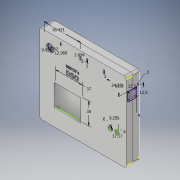
# Autodesk Inventor part: case
Saved by Autodesk Inventor 2019 (Build 230136000, 136)
## iProperties
Created: 2019-10-15
Part Number: case
Material: Generic
Document SubType Name: Modeling
Designer: Bill
Density: 1 g/cm^3
Appearance: Default
Author: Bill
Autodesk Inventor part; units mm, degrees
ref_plane "YZ Plane" through (0, 0, 0) normal (1, 0, 0) x (0, 1, 0)
ref_plane "XZ Plane" through (0, 0, 0) normal (0, 1, 0) x (-1, 0, 0)
ref_plane "XY Plane" through (0, 0, 0) normal (0, 0, 1) x (1, 0, 0)
sketch "Sketch1" plane through (0, 0, 0) normal (0, 0, 1) x (1, 0, 0)
  line L0 (0, 0) -> (110, 0) construction
  line L1 (110, 0) -> (110, 100) construction
  line L2 (110, 100) -> (0, 100) construction
  line L3 (0, 100) -> (0, 0) construction
  circle A0 centre (4, 96) radius 1.4
  circle A1 centre (106, 96) radius 1.4
  circle A2 centre (4, 4) radius 1.4
  circle A3 centre (106, 4) radius 1.4
  line L4 (-3, -3) -> (113, -3)
  line L5 (113, -3) -> (113, 103)
  line L6 (113, 103) -> (-3, 103)
  line L7 (-3, 103) -> (-3, -3)
  circle A4 centre (4, 96) radius 2
  circle A5 centre (106, 96) radius 2
  circle A6 centre (106, 4) radius 2
  circle A7 centre (4, 4) radius 2
  dimension "d0" = 100
  dimension "d1" = 110
  dimension "d2" = 2.8
  dimension "d3" = 2.8
  dimension "d4" = 2.8
  dimension "d5" = 2.8
  dimension "d6" = 4
  dimension "d7" = 4
  dimension "d8" = 4
  dimension "d9" = 4
  dimension "d10" = 4
  dimension "d11" = 4
  dimension "d12" = 4
  dimension "d13" = 4
  dimension "d14" = 3
  dimension "d27" = 4
  dimension "d28" = 4
  constraints: 16 end point, 8 centre point, 4 coincident, 4 parallel, 2 perpendicular, 1 horizontal, 3 other
  measures "d0" distance between parallel lines of L0 L2
  measures "d1" distance between parallel lines of L1 L3
  measures "d2" diameter of A0
  measures "d3" diameter of A1
  measures "d4" diameter of A2
  measures "d5" diameter of A3
  measures "d6" distance from line of L3 A0.centre
  measures "d7" distance from line of L2 A0.centre
  measures "d8" distance from line of A1.centre L2
  measures "d9" distance from line of L1 A1.centre
  measures "d10" distance from line of L3 A2.centre
  measures "d11" distance from line of L0 A2.centre
  measures "d12" distance from line of L1 A3.centre
  measures "d13" distance from line of L0 A3.centre
  measures "d14" distance between parallel lines of L3 L7
  measures "d27" diameter of A4
  measures "d28" diameter of A5
extrude "Extrusion1" add sketch "Sketch1" along normal blind 15 contours A0 | A1 | A2 | A3 | L7 L6 L5 L4 | A4 | A5 | A6 | A7
shell "Shell3" thickness 1.6 outward yes removed faces 0
ref_plane "Work Plane1" through (0, 0, 7.5) normal (0, 0, -1) x (-1, 0, 0)
split body "Split1" result two bodies by plane through (0, 0, 7.5) normal (0, 0, -1) first body at (74.8667, 68.2, -1.1)
extrude "Extrusion2" add sketch "Sketch1" along normal blind 10 contours A0 | A1 | A2 | A3 bodies 2
extrude "Extrusion3" add sketch "Sketch1" along normal blind 2 contours A4 | A5 | A6 | A7 bodies 2
fillet "Fillet1" radius 3 4 edges at (-4.6, -4.6, 12.05) (114.6, -4.6, 12.05) (113, 103, 11.25) (-4.6, 104.6, 12.05)
fillet "Fillet2" radius 3 4 edges at (-4.6, 104.6, 2.95) (114.6, 104.6, 2.95) (114.6, -4.6, 2.95) (-4.6, -4.6, 2.95)
fillet "Fillet3" radius 3 1 edges at (114.6, 104.6, 12.05)
ref_plane "Work Plane2" through (113, 103, 7.5) normal (0, 0, 1) x (1, 0, 0)
sketch "Sketch4" plane through (113, -3, 15) normal (0, 0, -1) x (-1, 0, 0)
  circle A0 centre (103.074, 90.001) radius 5.3099
  line L0 (116, 0) -> (116, 106) projected
  line L1 (116, 106) -> (0, 106) projected
  circle A1 centre (109, 99) radius 1.4 projected
  circle A2 centre (7, 99) radius 1.4 projected
  line L2 (3, 103) -> (113, 103) construction
  line L3 (3, 3) -> (3, 103) construction
  circle A3 centre (7, 7) radius 1.4 projected
  line L4 (113, 3) -> (3, 3) construction
  circle A4 centre (109, 7) radius 1.4 projected
  line L5 (113, 103) -> (113, 3) construction
  line L6 (62.579, 100.906) -> (60.579, 100.906)
  line L7 (60.579, 100.906) -> (60.579, 95.906)
  line L8 (60.579, 95.906) -> (62.579, 95.906)
  line L9 (62.579, 95.906) -> (62.579, 100.906)
  line L10 (29.851, 100.906) -> (27.851, 100.906)
  line L11 (27.851, 100.906) -> (27.851, 95.906)
  line L12 (27.851, 95.906) -> (29.851, 95.906)
  line L13 (29.851, 95.906) -> (29.851, 100.906)
  line L14 (97.7641, 51.5876) -> (60.7641, 51.5876)
  line L15 (60.7641, 51.5876) -> (60.7641, 21.5876)
  line L16 (60.7641, 21.5876) -> (97.7641, 21.5876)
  line L17 (97.7641, 21.5876) -> (97.7641, 51.5876)
  circle A5 centre (20.17, 35.2618) radius 3
  circle A6 centre (10.914, 35.2618) radius 3
  circle A7 centre (109, 99) radius 2.2006
  circle A8 centre (7, 99) radius 2.2006
  circle A9 centre (7, 7) radius 2.2006
  circle A10 centre (109, 7) radius 2.2006
  dimension "d35" = 10.6198
  dimension "d36" = 9.926
  dimension "d37" = 12.999
  dimension "d38" = 2
  dimension "d39" = 5
  dimension "d40" = 2.094
  dimension "d41" = 50.421
  dimension "d42" = 2
  dimension "d43" = 24.851
  dimension "d44" = 17.17
  dimension "d45" = 9.256
  dimension "d46" = 6
  dimension "d47" = 6
  dimension "d67" = 37
  dimension "d68" = 30
  constraints: 24 end point, 7 centre point, 6 parallel, 4 coincident, 3 horizontal, 3 perpendicular
  measures "d35" diameter of A0
  measures "d36" distance from line of L5 A0.centre
  measures "d37" distance from line of A0.centre L2
  measures "d38" distance between parallel lines of L7 L9
  measures "d39" distance between parallel lines of L8 L6
  measures "d40" distance between parallel lines of L6 L2
  measures "d41" distance between parallel lines of L5 L9
  measures "d42" distance of L12.end L11.end
  measures "d43" distance between parallel lines of L3 L11
  measures "d44" distance from line of L3 A5.centre
  measures "d45" distance of A6.centre A5.centre
  measures "d46" diameter of A5
  measures "d47" diameter of A6
  measures "d67" distance between parallel lines of L15 L17
  measures "d68" distance of L14.end L15.end
extrude "Extrusion4" add sketch "Sketch4" along normal blind 4 contours A7 | A8 | A9 | A10 bodies 3
extrude "Extrusion5" cut sketch "Sketch4" along normal mid plane 4 contours A0 | L9 L8 L7 L6 | L13 L12 L11 L10 | L17 L16 L15 L14 | A5 | A6 bodies 2
extrude "Extrusion6" cut sketch "Sketch4" against normal blind 3 contours A0 | L9 L8 L7 L6 | L13 L12 L11 L10 | L17 L16 L15 L14 | A5 | A6 bodies 3
sketch "Sketch5" plane through (114.6, -1.6, 16.6) normal (1, 0, 0) x (0, 0, -1)
  line L0 (3.7, 75.2) -> (12.2, 75.2)
  line L1 (14.2, 77.2) -> (14.2, 85.7)
  line L2 (12.2, 87.7) -> (3.7, 87.7)
  line L3 (1.7, 85.7) -> (1.7, 77.2)
  arc A0 (14.2, 85.7) -> (12.2, 87.7) centre (12.2, 85.7) ccw
  arc A1 (3.7, 87.7) -> (1.7, 85.7) centre (3.7, 85.7) ccw
  arc A2 (1.7, 77.2) -> (3.7, 75.2) centre (3.7, 77.2) ccw
  arc A3 (12.2, 75.2) -> (14.2, 77.2) centre (12.2, 77.2) ccw
  line L4 (18.2, 0) -> (18.2, 103.2) projected
  line L5 (9.1, 0) -> (0, 0) projected
  line L6 (0, 103.2) -> (9.1, 103.2) projected
  point P0 (16.6, 1.6)
  point P1 (14.2, 87.7)
  point P2 (1.7, 87.7)
  dimension "d55" = 12.5
  dimension "d56" = 12.5
  dimension "d57" = 2
  dimension "d58" = 4
  dimension "d64" = 15.5
  constraints: 8 end point, 8 point on circle, 8 tangent, 4 centre point, 4 point on line, 3 equal radius, 2 parallel, 1 horizontal, 1 perpendicular
  measures "d55" distance of point (1.7, 87.7) point (14.2, 87.7)
  measures "d56" distance between parallel lines of L0 L2
  measures "d57" radius of A0
  measures "d58" distance between parallel lines of L4 L1
  measures "d64" distance between parallel lines of L6 L2
extrude "Extrusion7" cut sketch "Sketch5" against normal blind 10 bodies 2
extrude "Extrusion8" cut sketch "Sketch5" against normal blind 10 bodies 3
sketch "Sketch6" plane through (0, 0, 16.6) normal (0, 0, 1) x (1, 0, 0)
  line L0 (31.2907, 78.1135) -> (77.2275, 78.1135) construction
  line L1 (77.2275, 78.1135) -> (77.2275, 50.5514) construction
  line L2 (77.2275, 50.5514) -> (31.2907, 50.5514) construction
  line L3 (31.2907, 50.5514) -> (31.2907, 78.1135) construction
  spline S0 degree 2 poles (34.1795, 75.7485) (34.1795, 75.5099) (33.998, 75.1495) (33.8476, 75.0302) knots 0 0 0 1 2 2 2
  spline S1 degree 2 poles (33.8476, 75.0302) (33.666, 74.8876) (33.2356, 74.7683) (32.901, 74.7683) knots 0 0 0 1 2 2 2
  line L4 (32.901, 74.7683) -> (31.6226, 74.7683)
  line L5 (31.6226, 74.7683) -> (31.6226, 77.9683)
  line L6 (31.6226, 77.9683) -> (32.7506, 77.9683)
  spline S2 degree 2 poles (32.7506, 77.9683) (33.1033, 77.9683) (33.4664, 77.9138) (33.6245, 77.8282) knots 0 0 0 1 2 2 2
  spline S3 degree 2 poles (33.6245, 77.8282) (33.7983, 77.7375) (33.9668, 77.4263) (33.9668, 77.224) knots 0 0 0 1 2 2 2
  spline S4 degree 2 poles (33.9668, 77.224) (33.9668, 76.9906) (33.7335, 76.625) (33.526, 76.5394) knots 0 0 0 1 2 2 2
  line L7 (33.526, 76.5394) -> (33.526, 76.5239)
  spline S5 degree 2 poles (33.526, 76.5239) (33.8242, 76.4616) (34.1795, 76.0752) (34.1795, 75.7485) knots 0 0 0 1 2 2 2
  spline S6 degree 2 poles (33.3497, 75.7615) (33.3497, 75.9119) (33.2304, 76.0804) (33.1111, 76.1245) knots 0 0 0 1 2 2 2
  spline S7 degree 2 poles (33.1111, 76.1245) (33.0385, 76.153) (32.7818, 76.1582) (32.5691, 76.1582) knots 0 0 0 1 2 2 2
  line L8 (32.5691, 76.1582) -> (32.4213, 76.1582)
  line L9 (32.4213, 76.1582) -> (32.4213, 75.3517)
  line L10 (32.4213, 75.3517) -> (32.4654, 75.3517)
  spline S8 degree 2 poles (32.4654, 75.3517) (32.7766, 75.3517) (33.0151, 75.3595) (33.1396, 75.414) knots 0 0 0 1 2 2 2
  spline S9 degree 2 poles (33.1396, 75.414) (33.2485, 75.4632) (33.3497, 75.6448) (33.3497, 75.7615) knots 0 0 0 1 2 2 2
  spline S10 degree 2 poles (33.15, 77.0658) (33.15, 77.1436) (33.0696, 77.307) (32.9866, 77.3433) knots 0 0 0 1 2 2 2
  spline S11 degree 2 poles (32.9866, 77.3433) (32.9088, 77.3796) (32.691, 77.3848) (32.4758, 77.3848) knots 0 0 0 1 2 2 2
  line L11 (32.4758, 77.3848) -> (32.4213, 77.3848)
  line L12 (32.4213, 77.3848) -> (32.4213, 76.7054)
  line L13 (32.4213, 76.7054) -> (32.5224, 76.7054)
  spline S12 degree 2 poles (32.5224, 76.7054) (32.7273, 76.7054) (32.8933, 76.7132) (32.9814, 76.7547) knots 0 0 0 1 2 2 2
  spline S13 degree 2 poles (32.9814, 76.7547) (33.0774, 76.8013) (33.15, 76.9595) (33.15, 77.0658) knots 0 0 0 1 2 2 2
  line L14 (35.349, 74.7683) -> (34.597, 74.7683)
  line L15 (34.597, 74.7683) -> (34.597, 77.1825)
  line L16 (34.597, 77.1825) -> (35.349, 77.1825)
  line L17 (35.349, 77.1825) -> (35.349, 74.7683)
  line L18 (35.3724, 77.5274) -> (34.5763, 77.5274)
  line L19 (34.5763, 77.5274) -> (34.5763, 78.1135)
  line L20 (34.5763, 78.1135) -> (35.3724, 78.1135)
  line L21 (35.3724, 78.1135) -> (35.3724, 77.5274)
  line L22 (36.6767, 74.7683) -> (35.9247, 74.7683)
  line L23 (35.9247, 74.7683) -> (35.9247, 78.1109)
  line L24 (35.9247, 78.1109) -> (36.6767, 78.1109)
  line L25 (36.6767, 78.1109) -> (36.6767, 74.7683)
  line L26 (38.0045, 74.7683) -> (37.2524, 74.7683)
  line L27 (37.2524, 74.7683) -> (37.2524, 78.1109)
  line L28 (37.2524, 78.1109) -> (38.0045, 78.1109)
  line L29 (38.0045, 78.1109) -> (38.0045, 74.7683)
  line L30 (41.2848, 77.9683) -> (40.1801, 76.1038)
  line L31 (40.1801, 76.1038) -> (40.1801, 74.7683)
  line L32 (40.1801, 74.7683) -> (39.3763, 74.7683)
  line L33 (39.3763, 74.7683) -> (39.3763, 76.0649)
  line L34 (39.3763, 76.0649) -> (38.2534, 77.9683)
  line L35 (38.2534, 77.9683) -> (39.1688, 77.9683)
  line L36 (39.1688, 77.9683) -> (39.7938, 76.8273)
  line L37 (39.7938, 76.8273) -> (40.398, 77.9683)
  line L38 (40.398, 77.9683) -> (41.2848, 77.9683)
  spline S14 degree 2 poles (43.1545, 75.707) (43.1545, 75.4995) (43.0119, 75.1313) (42.8693, 75.0017) knots 0 0 0 1 2 2 2
  spline S15 degree 2 poles (42.8693, 75.0017) (42.7085, 74.8564) (42.2703, 74.719) (41.985, 74.719) knots 0 0 0 1 2 2 2
  spline S16 degree 2 poles (41.985, 74.719) (41.7724, 74.719) (41.3989, 74.7501) (41.2563, 74.7812) knots 0 0 0 1 2 2 2
  line L39 (41.2563, 74.7812) -> (41.2563, 75.4295)
  line L40 (41.2563, 75.4295) -> (41.3289, 75.4295)
  spline S17 degree 2 poles (41.3289, 75.4295) (41.4249, 75.3906) (41.6349, 75.3232) (41.8009, 75.3232) knots 0 0 0 1 2 2 2
  spline S18 degree 2 poles (41.8009, 75.3232) (42.0135, 75.3232) (42.2443, 75.4425) (42.291, 75.5514) knots 0 0 0 1 2 2 2
  spline S19 degree 2 poles (42.291, 75.5514) (42.3403, 75.6577) (42.3506, 75.9326) (42.3506, 76.1038) knots 0 0 0 1 2 2 2
  line L41 (42.3506, 76.1038) -> (42.3506, 77.3874)
  line L42 (42.3506, 77.3874) -> (41.6194, 77.3874)
  line L43 (41.6194, 77.3874) -> (41.6194, 77.9683)
  line L44 (41.6194, 77.9683) -> (43.1545, 77.9683)
  line L45 (43.1545, 77.9683) -> (43.1545, 75.707)
  line L46 (44.3915, 74.7683) -> (44.3915, 77.3589)
  line L47 (44.3915, 77.3589) -> (43.445, 77.3589)
  line L48 (43.445, 77.3589) -> (43.445, 77.9683)
  line L49 (43.445, 77.9683) -> (46.1419, 77.9683)
  line L50 (46.1419, 77.9683) -> (46.1419, 77.3589)
  line L51 (46.1419, 77.3589) -> (45.1954, 77.3589)
  line L52 (45.1954, 77.3589) -> (45.1954, 74.7683)
  line L53 (45.1954, 74.7683) -> (44.3915, 74.7683)
  line L54 (47.0962, 78.1109) -> (46.9665, 76.8454)
  line L55 (46.9665, 76.8454) -> (46.5257, 76.8454)
  line L56 (46.5257, 76.8454) -> (46.396, 78.1109)
  line L57 (46.396, 78.1109) -> (47.0962, 78.1109)
  spline S20 degree 2 poles (48.372, 74.7034) (48.1075, 74.7034) (47.633, 74.8201) (47.4774, 74.8979) knots 0 0 0 1 2 2 2
  line L58 (47.4774, 74.8979) -> (47.4774, 75.5333)
  line L59 (47.4774, 75.5333) -> (47.5396, 75.5333)
  spline S21 degree 2 poles (47.5396, 75.5333) (47.5941, 75.4918) (47.7315, 75.3932) (47.8534, 75.3388) knots 0 0 0 1 2 2 2
  spline S22 degree 2 poles (47.8534, 75.3388) (47.9597, 75.2895) (48.2216, 75.2195) (48.3772, 75.2195) knots 0 0 0 1 2 2 2
  spline S23 degree 2 poles (48.3772, 75.2195) (48.5354, 75.2195) (48.7792, 75.318) (48.7792, 75.4243) knots 0 0 0 1 2 2 2
  spline S24 degree 2 poles (48.7792, 75.4243) (48.7792, 75.5073) (48.6677, 75.5955) (48.5069, 75.6318) knots 0 0 0 1 2 2 2
  spline S25 degree 2 poles (48.5069, 75.6318) (48.4213, 75.6551) (48.1594, 75.7044) (48.0583, 75.7355) knots 0 0 0 1 2 2 2
  spline S26 degree 2 poles (48.0583, 75.7355) (47.773, 75.8237) (47.4878, 76.1686) (47.4878, 76.4513) knots 0 0 0 1 2 2 2
  spline S27 degree 2 poles (47.4878, 76.4513) (47.4878, 76.612) (47.6356, 76.8973) (47.7808, 77.0088) knots 0 0 0 1 2 2 2
  spline S28 degree 2 poles (47.7808, 77.0088) (47.9234, 77.1177) (48.3461, 77.2474) (48.6132, 77.2474) knots 0 0 0 1 2 2 2
  spline S29 degree 2 poles (48.6132, 77.2474) (48.8673, 77.2474) (49.2926, 77.1462) (49.4378, 77.0762) knots 0 0 0 1 2 2 2
  line L60 (49.4378, 77.0762) -> (49.4378, 76.4642)
  line L61 (49.4378, 76.4642) -> (49.3782, 76.4642)
  spline S30 degree 2 poles (49.3782, 76.4642) (49.3393, 76.4953) (49.1707, 76.5965) (49.0929, 76.6328) knots 0 0 0 1 2 2 2
  spline S31 degree 2 poles (49.0929, 76.6328) (48.997, 76.6743) (48.7636, 76.7313) (48.6417, 76.7313) knots 0 0 0 1 2 2 2
  spline S32 degree 2 poles (48.6417, 76.7313) (48.4784, 76.7313) (48.2527, 76.6198) (48.2527, 76.529) knots 0 0 0 1 2 2 2
  spline S33 degree 2 poles (48.2527, 76.529) (48.2527, 76.4461) (48.3643, 76.3527) (48.551, 76.306) knots 0 0 0 1 2 2 2
  spline S34 degree 2 poles (48.551, 76.306) (48.6469, 76.2827) (48.8985, 76.2386) (49.0151, 76.1997) knots 0 0 0 1 2 2 2
  spline S35 degree 2 poles (49.0151, 76.1997) (49.2745, 76.1167) (49.5442, 75.7926) (49.5442, 75.5229) knots 0 0 0 1 2 2 2
  spline S36 degree 2 poles (49.5442, 75.5229) (49.5442, 75.3543) (49.386, 75.0457) (49.2382, 74.942) knots 0 0 0 1 2 2 2
  spline S37 degree 2 poles (49.2382, 74.942) (49.0852, 74.8279) (48.6651, 74.7034) (48.372, 74.7034) knots 0 0 0 1 2 2 2
  spline S38 degree 2 poles (37.366, 68.8889) (37.366, 68.0337) (36.6195, 66.6892) (36.051, 66.3283) knots 0 0 0 1 2 2 2
  spline S39 degree 2 poles (36.051, 66.3283) (35.5765, 66.0218) (34.4593, 65.8439) (33.8315, 65.8439) knots 0 0 0 1 2 2 2
  line L62 (33.8315, 65.8439) -> (31.9234, 65.8439)
  line L63 (31.9234, 65.8439) -> (31.9234, 71.9439)
  line L64 (31.9234, 71.9439) -> (33.8117, 71.9439)
  spline S40 degree 2 poles (33.8117, 71.9439) (34.4544, 71.9439) (35.5765, 71.7807) (36.0708, 71.4644) knots 0 0 0 1 2 2 2
  spline S41 degree 2 poles (36.0708, 71.4644) (36.669, 71.0788) (37.366, 69.7738) (37.366, 68.8889) knots 0 0 0 1 2 2 2
  spline S42 degree 2 poles (35.794, 68.8988) (35.794, 69.5019) (35.3788, 70.362) (34.9536, 70.6042) knots 0 0 0 1 2 2 2
  spline S43 degree 2 poles (34.9536, 70.6042) (34.6422, 70.7723) (33.96, 70.8069) (33.4855, 70.8069) knots 0 0 0 1 2 2 2
  line L65 (33.4855, 70.8069) -> (33.4558, 70.8069)
  line L66 (33.4558, 70.8069) -> (33.4558, 66.9858)
  line L67 (33.4558, 66.9858) -> (33.4855, 66.9858)
  spline S44 degree 2 poles (33.4855, 66.9858) (33.9996, 66.9858) (34.7065, 67.0204) (35.0278, 67.223) knots 0 0 0 1 2 2 2
  spline S45 degree 2 poles (35.0278, 67.223) (35.4035, 67.4603) (35.794, 68.2957) (35.794, 68.8988) knots 0 0 0 1 2 2 2
  spline S46 degree 2 poles (40.1589, 65.7351) (39.457, 65.7351) (38.3991, 66.007) (37.9443, 66.2047) knots 0 0 0 1 2 2 2
  line L68 (37.9443, 66.2047) -> (37.9443, 67.6581)
  line L69 (37.9443, 67.6581) -> (38.0827, 67.6581)
  spline S47 degree 2 poles (38.0827, 67.6581) (38.5425, 67.2675) (39.6448, 66.8474) (40.1639, 66.8474) knots 0 0 0 1 2 2 2
  spline S48 degree 2 poles (40.1639, 66.8474) (40.2973, 66.8474) (40.7274, 66.9067) (40.8559, 66.966) knots 0 0 0 1 2 2 2
  spline S49 degree 2 poles (40.8559, 66.966) (41.0141, 67.0352) (41.2365, 67.2873) (41.2365, 67.49) knots 0 0 0 1 2 2 2
  spline S50 degree 2 poles (41.2365, 67.49) (41.2365, 67.7223) (40.8757, 68.009) (40.6285, 68.0733) knots 0 0 0 1 2 2 2
  spline S51 degree 2 poles (40.6285, 68.0733) (40.3171, 68.1573) (39.6102, 68.3007) (39.2988, 68.4094) knots 0 0 0 1 2 2 2
  spline S52 degree 2 poles (39.2988, 68.4094) (38.5919, 68.6566) (37.9789, 69.5019) (37.9789, 70.1346) knots 0 0 0 1 2 2 2
  spline S53 degree 2 poles (37.9789, 70.1346) (37.9789, 70.9898) (39.4273, 72.0526) (40.5148, 72.0526) knots 0 0 0 1 2 2 2
  spline S54 degree 2 poles (40.5148, 72.0526) (41.0586, 72.0526) (42.1362, 71.8302) (42.5613, 71.6423) knots 0 0 0 1 2 2 2
  line L70 (42.5613, 71.6423) -> (42.5613, 70.2483)
  line L71 (42.5613, 70.2483) -> (42.4279, 70.2483)
  spline S55 degree 2 poles (42.4279, 70.2483) (42.0868, 70.54) (41.108, 70.9404) (40.5939, 70.9404) knots 0 0 0 1 2 2 2
  spline S56 degree 2 poles (40.5939, 70.9404) (40.3912, 70.9404) (40.0749, 70.8811) (39.8969, 70.802) knots 0 0 0 1 2 2 2
  spline S57 degree 2 poles (39.8969, 70.802) (39.7536, 70.7377) (39.5459, 70.4807) (39.5459, 70.3225) knots 0 0 0 1 2 2 2
  spline S58 degree 2 poles (39.5459, 70.3225) (39.5459, 70.0852) (39.8771, 69.8133) (40.3517, 69.7046) knots 0 0 0 1 2 2 2
  spline S59 degree 2 poles (40.3517, 69.7046) (40.6582, 69.6354) (41.2267, 69.5019) (41.5529, 69.3882) knots 0 0 0 1 2 2 2
  spline S60 degree 2 poles (41.5529, 69.3882) (42.1857, 69.1559) (42.8036, 68.3847) (42.8036, 67.752) knots 0 0 0 1 2 2 2
  spline S61 degree 2 poles (42.8036, 67.752) (42.8036, 66.8424) (41.375, 65.7351) (40.1589, 65.7351) knots 0 0 0 1 2 2 2
  spline S62 degree 2 poles (49.1408, 68.8939) (49.1408, 67.4109) (47.559, 65.7153) (46.1848, 65.7153) knots 0 0 0 1 2 2 2
  spline S63 degree 2 poles (46.1848, 65.7153) (44.8056, 65.7153) (43.2336, 67.4307) (43.2336, 68.8939) knots 0 0 0 1 2 2 2
  spline S64 degree 2 poles (43.2336, 68.8939) (43.2336, 70.362) (44.8056, 72.0724) (46.1848, 72.0724) knots 0 0 0 1 2 2 2
  spline S65 degree 2 poles (46.1848, 72.0724) (47.559, 72.0724) (49.1408, 70.3719) (49.1408, 68.8939) knots 0 0 0 1 2 2 2
  spline S66 degree 2 poles (47.559, 68.8939) (47.559, 69.4426) (47.3365, 70.2088) (47.1438, 70.451) knots 0 0 0 1 2 2 2
  spline S67 degree 2 poles (47.1438, 70.451) (46.951, 70.7031) (46.4566, 70.9206) (46.1897, 70.9206) knots 0 0 0 1 2 2 2
  spline S68 degree 2 poles (46.1897, 70.9206) (45.9079, 70.9206) (45.4482, 70.7179) (45.2357, 70.4609) knots 0 0 0 1 2 2 2
  spline S69 degree 2 poles (45.2357, 70.4609) (45.0478, 70.2236) (44.8155, 69.4376) (44.8155, 68.8939) knots 0 0 0 1 2 2 2
  spline S70 degree 2 poles (44.8155, 68.8939) (44.8155, 68.3303) (45.0379, 67.5888) (45.2307, 67.3367) knots 0 0 0 1 2 2 2
  spline S71 degree 2 poles (45.2307, 67.3367) (45.4235, 67.0846) (45.9228, 66.8671) (46.1897, 66.8671) knots 0 0 0 1 2 2 2
  spline S72 degree 2 poles (46.1897, 66.8671) (46.4616, 66.8671) (46.9658, 67.0995) (47.1487, 67.3466) knots 0 0 0 1 2 2 2
  spline S73 degree 2 poles (47.1487, 67.3466) (47.3464, 67.6136) (47.559, 68.3205) (47.559, 68.8939) knots 0 0 0 1 2 2 2
  point P0 (0, 0)
  constraints: 2 other
extrude "Extrusion9" cut sketch "Sketch6" against normal blind 3 bodies 3
body "Solid2"
body "Solid3"
